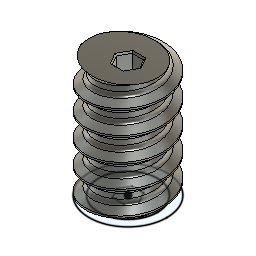
Corkscrew Roller (Autodesk Fusion 360 design; units mm, degrees)
Autodesk Fusion 360 part; units mm, degrees
note: some values were not read from the file. Chosen so that the rebuilt part matches the saved one: which face or edge a step refers to.
sketch "Sketch9" plane through (0, 0, 0) normal (0, 0, 1) x (1, 0, 0)
  circle A0 centre (0, 0) radius 19.05
  circle A1 centre (0, 0) radius 25.4
  circle A2 centre (0, 0) radius 19.304
  line L0 (-3.7395, 6.477) -> (-7.479, 0)
  line L1 (-7.479, 0) -> (-3.7395, -6.477)
  line L2 (-3.7395, -6.477) -> (3.7395, -6.477)
  line L3 (3.7395, -6.477) -> (7.479, 0)
  line L4 (7.479, 0) -> (3.7395, 6.477)
  line L5 (3.7395, 6.477) -> (-3.7395, 6.477)
  dimension "d21" = 38.1
  dimension "d22" = 50.8
  dimension "d31" = 38.608
  dimension "d36" = 6.477
  constraint coincident A0.centre A1.centre
  constraint concentric A0 A1
  constraint concentric A1 A2
  constraint horizontal L5
  measures "d21" diameter of A0
  measures "d22" diameter of A1
  measures "d31" diameter of A2
  measures "d36" distance of A0.centre L5
extrude "Extrude2" add sketch "Sketch9" along normal blind 76.2 contours A0 | A1 | A2
ref_plane "WorkPlane3" through (0, 0, -15.24) normal (0, 0, 1) x (1, 0, 0)
coil "CoilPrimitive2" cut diameter 50.8 section triangle in size 12.192 inside turns 7 pitch 15.24 right hand placed x (1, 0, 0) y (0, 1, 0) z (0, 0, 1) at (0, 0, -15.24)
extrude "Extrude3" add sketch "Sketch9" along normal blind 76.2 contours A0 | A2
fillet "Fillet1" radius 3.175 22 edges at (14.4423, -12.8088, 1.7598) (0, 19.304, 7.3295) (0, -19.304, 14.9495) (0, -19.304, 7.9105) (-12.8088, 14.4423, 2.0502) (0, 19.304, 61.2505) (0, 19.304, 68.2895) (-12.8088, -14.4423, 74.1498) (0, -19.304, 68.8705) (14.4423, 12.8088, 74.4402) (0, 19.304, 15.5305) (0, 19.304, 22.5695) (0, -19.304, 30.1895) (0, -19.304, 23.1505) (0, 19.304, 46.0105) (0, 19.304, 53.0495) (0, -19.304, 60.6695) (0, -19.304, 53.6305) (0, 19.304, 30.7705) (0, 19.304, 37.8095) (0, -19.304, 45.4295) (0, -19.304, 38.3905)
chamfer "Chamfer1" distance 0.9 angle 45 12 edges at (0, 6.477, 76.2) (5.6092, 3.2385, 76.2) (5.6092, -3.2385, 76.2) (0, -6.477, 76.2) (-5.6092, -3.2385, 76.2) (-5.6092, 3.2385, 76.2) (5.6092, -3.2385, 0) (0, -6.477, 0) (-5.6092, -3.2385, 0) (-5.6092, 3.2385, 0) (0, 6.477, 0) (5.6092, 3.2385, 0)
equation "ID = 1.5 in"
equation "ROOT = ID + 0.02 in"
equation "OD = 2 in"
equation "PITCH = 0.6 in"
equation "TURNS = 5"
equation "d21 = ID"
equation "d22 = OD"
equation "d23 = PITCH * TURNS"
equation "d25 = -PITCH"
equation "d26 = OD"
equation "d27 = ( OD - ROOT )"
equation "d29 = TURNS + 2"
equation "d30 = PITCH"
equation "d31 = ROOT"
equation "d32 = PITCH * TURNS"
equation "d36 = 0.51 in / 2"
